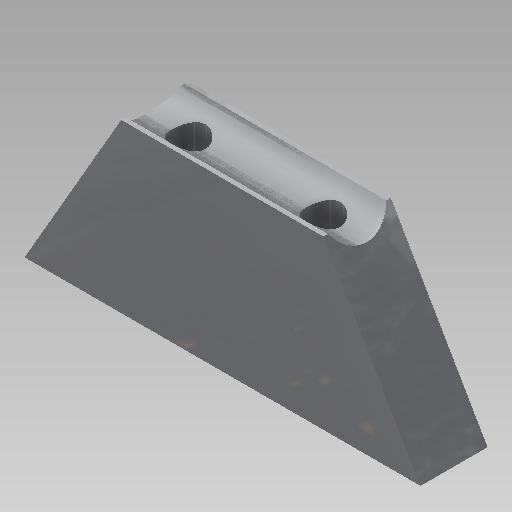
# Autodesk Inventor part: PWTR-0039
Saved by Autodesk Inventor 2020 (Build 240168000, 168)
## iProperties
Part Number: PWTR-0039
Document SubType Name: Modeling
Created: 2003-02-05
Designer: B. BOGAN
Description: TROWEL STANDOFF
Material: Aluminum-6061
Density: 2.7 g/cm^3
Appearance: Aluminum - Flat
Mass: 53.8548 g
Surface Area: 70.1515 cm^2
Volume: 19.9462 cm^3
Vendor: Non-Design Specific
Control State: 0
Master: False
Checked Out: False
Shininess: 64.0
Length Units: 11269
Angle Units: 11279
Time Units: 11290
Mass Units: 11283
Length Display Precision: 3
Angle Display Precision: 2
Compacted: True
Density: 0.0
Volumn: 0.0
Area: 0.0
PropertySet Name: Model Information
Title: TROWEL STANDOFF
Author: B. BOGAN
Revision Number: B
Autodesk Inventor part; units mm, degrees
ref_plane "YZ Plane" through (0, 0, 0) normal (1, 0, 0) x (0, 1, 0)
ref_plane "XZ Plane" through (0, 0, 0) normal (0, 1, 0) x (-1, 0, 0)
sketch "Sketch1" plane through (0, 0, 0) normal (0, 0, 1) x (1, 0, 0)
  line L0 (0, 0) -> (38.1, 0)
  line L1 (38.1, 0) -> (56.4309, -31.75)
  line L2 (56.4309, -31.75) -> (-18.3309, -31.75)
  line L3 (-18.3309, -31.75) -> (0, 0)
  dimension "d0" = 38.1
  dimension "d1" = 60
  dimension "d2" = 31.75
  constraints: 8 end point, 1 coincident, 1 equal length, 1 horizontal, 1 parallel
  measures "d0" distance of L0.start L0.end
  measures "d1" angle of L1 L2
  measures "d2" distance between parallel lines of L0 L2
extrude "Extrusion1" add sketch "Sketch1" along normal blind 12.7
ref_plane "Work Plane1" through (-3.175, 0, 0) normal (1, 0, 0) x (0, 1, 0)
sketch "Sketch2" plane through (-3.175, 0, 0) normal (1, 0, 0) x (0, 1, 0)
  line L0 (0, 0) -> (0, 12.7)
  circle A0 centre (3.175, 6.35) radius 6.35
  dimension "d5" = 3.175
  dimension "d6" = 12.7
  dimension "d7" = 9.525
  constraints: 2 end point, 1 centre point
  measures "d5" distance from line of A0.centre L0
  measures "d6" diameter of A0
extrude "Extrusion2" cut sketch "Sketch2" along normal through all
sketch "Sketch3" plane through (-18.3309, -31.75, 0) normal (0, -1, 0) x (1, 0, 0)
  line L0 (74.7617, 12.7) -> (0, 12.7) projected
  line L1 (74.7617, 0) -> (0, 0) projected
  line L2 (74.7617, 0) -> (74.7617, 12.7) projected
  line L3 (37.3809, 12.7) -> (37.3809, 0) construction
  line L4 (0.4848, 6.35) -> (74.7617, 6.35) construction
  point P0 (24.6809, 6.35)
  point P1 (50.0809, 6.35)
  dimension "d11" = 12.7
  dimension "d12" = 25.4
  constraints: 4 end point, 3 midpoint, 2 point on line
  measures "d11" distance from line of point (24.681, 6.35) L3
  measures "d12" distance of point (50.081, 6.35) point (24.681, 6.35)
hole "Hole1" at (6.35, -31.75, 6.35) at (31.75, -31.75, 6.35) direction (0, 1, 0) diameter 6.35 end through all
chamfer "Chamfer1" distance 0.2 angle 45 4 edges at (19.05, -31.75, 12.7) (-18.3309, -31.75, 6.35) (19.05, -31.75, 0) (56.4309, -31.75, 6.35)
body "Solid1"
